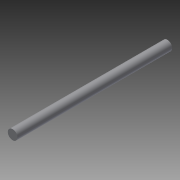
# Autodesk Inventor part: dead_axle
Saved by Autodesk Inventor 2015 SP1 (Build 190203100, 203)
## iProperties
Created: 2014-12-28
Part Number: dead_axle
Material: Generic
Document SubType Name: Modeling
Designer: Jarod
Density: 1 g/cm^3
Appearance: Default
Author: Jarod
Autodesk Inventor part; units mm, degrees
ref_plane "YZ Plane" through (0, 0, 0) normal (1, 0, 0) x (0, 1, 0)
ref_plane "XZ Plane" through (0, 0, 0) normal (0, 1, 0) x (-1, 0, 0)
ref_plane "XY Plane" through (0, 0, 0) normal (0, 0, 1) x (1, 0, 0)
sketch "Sketch1" plane through (0, 0, 0) normal (0, 0, 1) x (1, 0, 0)
  circle A0 centre (0, 0) radius 4.7625
  dimension "d0" = 9.525
  constraints: 1 centre point, 1 coincident
  measures "d0" diameter of A0
extrude "Extrusion1" add sketch "Sketch1" along normal blind 139.7
sketch "Sketch2" plane through (0, 0, 139.7) normal (0, 0, 1) x (1, 0, 0)
  circle A0 centre (0, 0) radius 4.7625 projected
  line L0 (0, 0) -> (0, 7.1437) construction
  line L1 (0, 0) -> (4.1244, 7.1437) construction
  line L2 (0, 0) -> (8.2489, 0) construction
  line L3 (4.1244, 7.1437) -> (-4.1244, 7.1437) construction
  line L4 (0, 0) -> (-4.1244, 7.1438) construction
  line L5 (-4.1244, 7.1438) -> (-8.2489, 0) construction
  line L6 (0, 0) -> (-8.2489, 0) construction
  line L7 (-8.2489, 0) -> (-4.1244, -7.1437) construction
  line L8 (0, 0) -> (-4.1244, -7.1437) construction
  line L9 (-4.1244, -7.1437) -> (4.1244, -7.1437) construction
  line L10 (0, 0) -> (4.1244, -7.1438) construction
  line L11 (4.1244, -7.1438) -> (8.2489, 0) construction
  line L12 (0, 0) -> (8.2489, 0) construction
  line L13 (8.2489, 0) -> (4.1244, 7.1437) construction
  line L14 (-4.1244, 7.1438) -> (4.1244, 7.1437)
  line L15 (4.1244, 7.1437) -> (8.2489, 0)
  line L16 (8.2489, 0) -> (4.1244, -7.1438)
  line L17 (4.1244, -7.1438) -> (-4.1244, -7.1437)
  line L18 (-4.1244, -7.1437) -> (-8.2489, 0)
  line L19 (-8.2489, 0) -> (-4.1244, 7.1438)
  dimension "d3" = 7.1437
  dimension "d4" = 60
  dimension "d7" = 360
  constraints: 40 end point, 3 equal length, 2 horizontal, 1 vertical, 31 other
  measures "d3" distance of L0.start L0.end
  measures "d4" angle of L2 L1
extrude "Extrusion2" add sketch "Sketch2" along normal blind 4.6355 contours A0 | L14 L15 L16 L17 L18 L19
body "Solid1"
